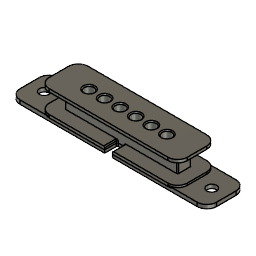
main (Autodesk Fusion 360 archive; units mm, degrees)
design "pickup_bobin"
Autodesk Fusion 360 part; units mm, degrees
sketch "Sketch1" plane through (0, 0, 0) normal (0, 0, 1) x (1, 0, 0)
  line L0 (5, 0) -> (66, 0)
  line L1 (71, 5) -> (71, 15)
  line L2 (66, 20) -> (5, 20)
  line L3 (0, 15) -> (0, 5)
  arc A0 (5, 20) -> (0, 15) centre (5, 15) ccw
  arc A1 (0, 5) -> (5, 0) centre (5, 5) ccw
  arc A2 (66, 0) -> (71, 5) centre (66, 5) ccw
  arc A3 (71, 15) -> (66, 20) centre (66, 15) ccw
  circle A4 centre (15.5, 10) radius 2.5
  circle A5 centre (23.5, 10) radius 2.5
  circle A6 centre (31.5, 10) radius 2.5
  circle A7 centre (39.5, 10) radius 2.5
  circle A8 centre (47.5, 10) radius 2.5
  circle A9 centre (55.5, 10) radius 2.5
  line L4 (7, 6.5) -> (64, 6.5)
  line L5 (64.5, 7) -> (64.5, 13)
  line L6 (64, 13.5) -> (7, 13.5)
  line L7 (6.5, 13) -> (6.5, 7)
  arc A10 (7, 13.5) -> (6.5, 13) centre (7, 13) ccw
  arc A11 (6.5, 7) -> (7, 6.5) centre (7, 7) ccw
  arc A12 (64, 6.5) -> (64.5, 7) centre (64, 7) ccw
  arc A13 (64.5, 13) -> (64, 13.5) centre (64, 13) ccw
  point P0 (71, 0)
  point P1 (0, 20)
  dimension "d11" = 71
  dimension "d12" = 20
  dimension "d13" = 5
  dimension "d14" = 5
  dimension "d17" = 5
  dimension "d19" = 8
  dimension "d20" = 5
  dimension "d21" = 5
  dimension "d22" = 5
  dimension "d23" = 5
  dimension "d24" = 8
  dimension "d25" = 8
  dimension "d26" = 8
  dimension "d27" = 8
  dimension "d33" = 10
  dimension "d34" = 10
  dimension "d37" = 6.5
  dimension "d38" = 6.5
  dimension "d39" = 6.5
  dimension "d40" = 6.5
  dimension "d41" = 0.5
  dimension "d52" = 15.5
  constraint horizontal L0
  constraint vertical L1
  constraint horizontal L2
  constraint vertical L3
  constraint coincident P1 L2
  constraint coincident P1 L3
  constraint tangent L2 A0
  constraint tangent L3 A0
  constraint coincident origin L0
  constraint coincident origin L3
  constraint tangent L0 A1
  constraint tangent L3 A1
  constraint equal A0 A1
  constraint coincident P0 L0
  constraint coincident P0 L1
  constraint tangent L0 A2
  constraint tangent L1 A2
  constraint equal A0 A2
  constraint tangent L1 A3
  constraint tangent L2 A3
  constraint equal A0 A3
  constraint collinear A4.centre A5.centre A6.centre
  constraint collinear A5.centre A6.centre A7.centre
  constraint collinear A6.centre A7.centre A8.centre
  constraint collinear A7.centre A8.centre A9.centre
  constraint horizontal L4
  constraint vertical L5
  constraint horizontal L6
  constraint vertical L7
  constraint tangent L6 A10
  constraint tangent L7 A10
  constraint tangent L4 A11
  constraint tangent L7 A11
  constraint equal A10 A11
  constraint tangent L4 A12
  constraint tangent L5 A12
  constraint equal A10 A12
  constraint tangent L5 A13
  constraint tangent L6 A13
  constraint equal A10 A13
  measures "d11" distance of origin P0
  measures "d12" distance of origin P1
  measures "d13" radius of A0
  measures "d14" diameter of A4
  measures "d17" diameter of A5
  measures "d19" distance of A4.centre A5.centre
  measures "d20" diameter of A6
  measures "d21" diameter of A7
  measures "d22" diameter of A8
  measures "d23" diameter of A9
  measures "d24" distance of A5.centre A6.centre
  measures "d25" distance of A6.centre A7.centre
  measures "d26" distance of A7.centre A8.centre
  measures "d27" distance of A8.centre A9.centre
  measures "d33" distance of L0 A4.centre
  measures "d34" distance of L0 A9.centre
  measures "d37" distance of L0 L4
  measures "d38" distance of L2 L6
  measures "d39" distance of L3 L7
  measures "d40" distance of L1 L5
  measures "d41" radius of A10
  measures "d52" distance of L1 A9.centre
extrude "Extrude1" add sketch "Sketch1" along normal blind 1.5 contours L0 L1 L2 L3 A0 A1 A2 A3 makes body 1
extrude "Extrude3" add sketch "Sketch1" against normal blind 1.5 from surface at 13 separate body contours L0 L1 L2 L3 A0 A1 A2 A3 makes body 2
extrude "Extrude2" add sketch "Sketch1" along normal blind 13 contours L4 L5 L6 L7 A10 A11 A12 A13 bodies 1 2
chamfer "Chamfer2" distance 0.5 angle 45 12 edges at (53.1692, 10.904, 13) (45.1692, 10.904, 13) (37.1692, 10.904, 13) (29.1692, 10.904, 13) (21.1692, 10.904, 13) (13.1692, 10.904, 13) (53.1692, 10.904, 0) (45.1692, 10.904, 0) (37.1692, 10.904, 0) (29.1692, 10.904, 0) (21.1692, 10.904, 0) (13.1692, 10.904, 0) on bodies 1
sketch "Sketch2" plane through (0, 0, 0) normal (0, 0, 1) x (1, 0, 0)
  line L0 (-10, 20) -> (81, 20)
  line L1 (86, 15) -> (86, 5)
  line L2 (81, 0) -> (-10, 0)
  line L3 (-15, 5) -> (-15, 15)
  arc A0 (-10, 20) -> (-15, 15) centre (-10, 15) ccw
  arc A1 (-15, 5) -> (-10, 0) centre (-10, 5) ccw
  arc A2 (81, 0) -> (86, 5) centre (81, 5) ccw
  arc A3 (86, 15) -> (81, 20) centre (81, 15) ccw
  circle A4 centre (-7.5, 10) radius 2.5
  circle A5 centre (78.5, 10) radius 2.5
  circle A6 centre (23.5, 10) radius 3
  circle A7 centre (39.5, 10) radius 3
  circle A8 centre (55.5, 10) radius 3
  arc A9 (71, 15) -> (66, 20) centre (66, 15) ccw
  line L4 (71, 15) -> (71, 5)
  arc A10 (66, 0) -> (71, 5) centre (66, 5) ccw
  line L5 (66, 0) -> (5, 0)
  arc A11 (0, 5) -> (5, 0) centre (5, 5) ccw
  line L6 (0, 5) -> (0, 15)
  arc A12 (5, 20) -> (0, 15) centre (5, 15) ccw
  line L7 (5, 20) -> (66, 20)
  circle A13 centre (47.5, 10) radius 3
  circle A14 centre (31.5, 10) radius 3
  circle A15 centre (15.5, 10) radius 3
  line L8 (15.5, 7) -> (55.5, 7)
  arc A16 (55.5, 7) -> (55.5, 13) centre (55.5, 10) ccw
  line L9 (55.5, 13) -> (15.5, 13)
  arc A17 (15.5, 13) -> (15.5, 7) centre (15.5, 10) ccw
  line L10 (15.5, 10) -> (55.5, 10) construction
  line L11 (33.5, 0) -> (37.5, 0)
  line L12 (37.5, 0) -> (37.5, 6.5)
  line L13 (37.5, 6.5) -> (33.5, 6.5)
  line L14 (33.5, 6.5) -> (33.5, 0)
  point P0 (-15, 20)
  point P1 (86, 20)
  point P2 (-15, 0)
  dimension "d55" = 101
  dimension "d56" = 20
  dimension "d57" = 5
  dimension "d58" = 10
  dimension "d59" = 7.5
  dimension "d60" = 7.5
  dimension "d61" = 10
  dimension "d68" = 6
  dimension "d69" = 4
  dimension "d70" = 6.5
  dimension "d71" = 33.5
  dimension "d86" = 15
  constraint horizontal L0
  constraint vertical L1
  constraint horizontal L2
  constraint vertical L3
  constraint coincident P0 L0
  constraint coincident P0 L3
  constraint tangent L0 A0
  constraint tangent L3 A0
  constraint coincident P2 L2
  constraint coincident P2 L3
  constraint tangent L2 A1
  constraint tangent L3 A1
  constraint equal A0 A1
  constraint tangent L1 A2
  constraint tangent L2 A2
  constraint equal A0 A2
  constraint coincident P1 L0
  constraint coincident P1 L1
  constraint tangent L0 A3
  constraint tangent L1 A3
  constraint equal A0 A3
  constraint tangent L8 A16
  constraint tangent A16 L9
  constraint parallel L8 L9
  constraint tangent L9 A17
  constraint tangent L8 A17
  constraint coincident A8.centre A16.centre
  constraint horizontal L10
  constraint coincident A15.centre A17.centre
  constraint horizontal L11
  constraint vertical L12
  constraint horizontal L13
  constraint vertical L14
  constraint coincident L2 L11.start
  measures "d55" distance of P0 P1
  measures "d56" distance of P0 P2
  measures "d57" radius of A0
  measures "d58" distance of L2 A5.centre
  measures "d59" distance of L1 A5.centre
  measures "d60" distance of L3 A4.centre
  measures "d61" distance of L2 A4.centre
  measures "d68" diameter of A16
  measures "d69" distance of L11.start L11.end
  measures "d70" distance of L11.start L13.end
  measures "d71" distance of L6 L14
  measures "d86" distance of L3 L6
extrude "Extrude4" add sketch "Sketch2" against normal blind 1.5 separate body makes body 3
extrude "Extrude6" add sketch "Sketch2" along normal blind 0.5 contours L0 L2 L3 A0 A1 A11 L6 A12 | L0 L1 L2 A2 A3 A9 L4 A10 bodies 3
extrude "Extrude7" cut sketch "Sketch2" along normal blind 1.5 contours L2 L5 L11 L12 L13 L14 bodies 1
extrude "Extrude8" cut sketch "Sketch2" against normal blind 1.5 contours L2 L5 L11 L12 L13 L14 bodies 3
fillet "Fillet2" radius 0.5 4 edges at (33.5, 6.5, 0.75) (37.5, 6.5, 0.75) (33.5, 6.5, -0.75) (37.5, 6.5, -0.75) on bodies 1 3
fillet "Fillet3" radius 0.5 4 edges at (37.3536, 6.3536, 1.5) (37.5, 3, 1.5) (33.5, 3, 1.5) (33.6464, 6.3536, 1.5) on bodies 1
extrude "Extrude9" add 1 faces at (36, 6.5, -0.5) along direction (0, 1, 0) blind 6.5 on bodies 3 bodies 3
fillet "Fillet4" radius 0.5 2 edges at (37, 7, -0.75) (34, 7, -0.75) on bodies 3
equation "magnet_diameter = 5 mm"
equation "pole_spacing = 8 mm"
equation "coil_width = 6.5 mm"
equation "bobin_length = 71 mm"
equation "bobin_width = 20 mm"
equation "flange_thickness = 1.5 mm"
equation "edge_radius = 0.5 mm"
equation "d11 = bobin_length"
equation "d12 = bobin_width"
equation "d13 = bobin_width / 4"
equation "d14 = magnet_diameter"
equation "d17 = magnet_diameter"
equation "d19 = pole_spacing"
equation "d20 = magnet_diameter"
equation "d21 = magnet_diameter"
equation "d22 = magnet_diameter"
equation "d23 = magnet_diameter"
equation "d24 = pole_spacing"
equation "d25 = pole_spacing"
equation "d26 = pole_spacing"
equation "d27 = pole_spacing"
equation "d33 = bobin_width / 2"
equation "d34 = bobin_width / 2"
equation "d37 = coil_width"
equation "d38 = coil_width"
equation "d39 = coil_width"
equation "d40 = coil_width"
equation "d41 = edge_radius"
equation "d42 = flange_thickness"
equation "d44 = bobin_height"
equation "d46 = bobin_height"
equation "d47 = -flange_thickness"
equation "magnet_length = 18 mm"
equation "bobin_height = magnet_length - 5 mm"
equation "outer_hole_spacing = ( bobin_length - 5 * pole_spacing ) / 2"
equation "d52 = outer_hole_spacing"
equation "d54 = edge_radius"
equation "d55 = 30 mm + bobin_length"
equation "d56 = bobin_width"
equation "d57 = bobin_width / 4"
equation "d58 = bobin_width / 2"
equation "d61 = bobin_width / 2"
equation "d62 = -flange_thickness"
equation "d68 = magnet_diameter + 1 mm"
equation "d70 = coil_width"
equation "d71 = ( bobin_length - 4 mm ) / 2"
equation "d72 = flange_thickness"
equation "d79 = edge_radius"
equation "d81 = edge_radius"
equation "d85 = edge_radius"
named bodies: "Pickup", "Mount"
